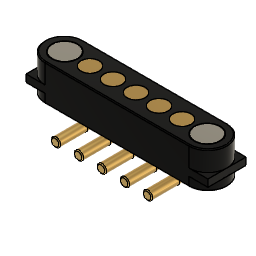
5359 Mag Connector (5-pin, Right Angle, Pads) (Autodesk Fusion 360 design; units mm, degrees)
Autodesk Fusion 360 part; units mm, degrees
sketch "Profile" plane through (0, 0, 0) normal (0, 0, 1) x (1, 0, 0)
  line L0 (-7.865, 0) -> (7.865, 0) construction
  line L1 (0, 2.1) -> (0, -2.1) construction
  circle A0 centre (-7.865, 0) radius 1.425
  line L2 (-10.04, 2.1) -> (10.04, 2.1)
  line L3 (10.04, 2.1) -> (10.04, -2.1)
  line L4 (10.04, -2.1) -> (-10.04, -2.1)
  line L5 (-10.04, -2.1) -> (-10.04, 2.1)
  circle A1 centre (-5.08, 0) radius 0.45
  circle A2 centre (-2.54, 0) radius 0.45
  circle A3 centre (0, 0) radius 0.45
  circle A4 centre (2.54, 0) radius 0.45
  circle A5 centre (5.08, 0) radius 0.45
  circle A6 centre (7.865, 0) radius 1.425
  arc A7 (-7.94, 2.1) -> (-7.94, -2.1) centre (-7.94, 0) ccw
  line L6 (-7.94, 2.1) -> (-7.94, -2.1) construction
  arc A8 (7.94, -2.1) -> (7.94, 2.1) centre (7.94, 0) ccw
  circle A9 centre (-5.08, 0) radius 0.5
  circle A10 centre (-5.08, 0) radius 1
  circle A11 centre (-2.54, 0) radius 0.5
  circle A12 centre (-2.54, 0) radius 1
  circle A13 centre (0, 0) radius 0.5
  circle A14 centre (0, 0) radius 1
  circle A15 centre (2.54, 0) radius 0.5
  circle A16 centre (2.54, 0) radius 1
  circle A17 centre (5.08, 0) radius 0.5
  circle A18 centre (5.08, 0) radius 1
  circle A19 centre (-5.08, 0) radius 0.575
  circle A20 centre (-2.54, 0) radius 0.575
  circle A21 centre (0, 0) radius 0.575
  circle A22 centre (2.54, 0) radius 0.575
  circle A23 centre (5.08, 0) radius 0.575
  dimension "d1" = 2.85
  dimension "d2" = 2.175
  dimension "d3" = 4.2
  dimension "d4" = 20.08
  dimension "d10" = 0.9
  dimension "d11" = 2.785
  dimension "d16" = 2.54
  dimension "d17" = 0
  dimension "d18" = 2.785
  dimension "d19" = 1
  dimension "d20" = 2
  dimension "d45" = 1.15
  constraint horizontal L0
  constraint coincident A3.centre L0
  constraint vertical L1
  constraint coincident L0 A0.centre
  constraint coincident L0.start A0.centre
  constraint horizontal L2
  constraint vertical L3
  constraint horizontal L4
  constraint vertical L5
  constraint symmetric L1 L3 L5
  constraint coincident L1.start L2
  constraint coincident L1.end L4
  constraint coincident L0 A1.centre
  constraint symmetric L1 A0 A6
  constraint coincident L2 A7.start
  constraint vertical L6
  constraint coincident L4 A7.end
  constraint coincident A7.centre L6
  constraint tangent L5 A7
  constraint symmetric L1 A7.start A8.end
  constraint symmetric L1 A7.end A8.start
  constraint symmetric L1 A7 A8
  constraint concentric A1 A9
  constraint concentric A1 A10
  constraint midpoint A3.centre L1
  constraint midpoint L0 A3.centre
  constraint concentric A10 A19
  measures "d1" diameter of A0
  measures "d2" distance of L0.start L5
  measures "d3" distance of L2.start L4.end
  measures "d4" distance of L2.start L2.end
  measures "d10" diameter of A1
  measures "d11" distance of L0.start A1.centre
  measures "d18" distance of A5.centre L0.end
  measures "d19" diameter of A9
  measures "d20" diameter of A10
  measures "d45" diameter of A19
extrude "Extrude - Housing" add sketch "Profile" along normal blind 4 contours L2 L4 A7 A8 makes body 1
extrude "Extrude - Housing Tabs" add sketch "Profile" along normal blind 0.8 from surface at 1 contours L2 L5 A7 | L4 L5 A7 | L2 L3 A8 | L3 L4 A8 bodies 1
fillet "Fillet - Housing Edges" radius 0.1 8 edges at (0, -2.1, 4) (10.04, 0, 4) (0, 2.1, 4) (-10.04, 0, 4) (0, -2.1, 0) (10.04, 0, 0) (0, 2.1, 0) (-10.04, 0, 0) on bodies 1
extrude "Extrude - Housing Pin Clearance" add sketch "Profile" along normal up to surface (3.8 mm away) from surface at 0.2 contours A10 | A12 | A14 | A16 | A18 bodies 1
copy_body "Body->Comp1" bodies 1 removing the originals makes body 2 in component "Housing"
extrude "Extrude - Magnets" add sketch "Profile" along normal blind 4 separate body contours A0 | A6 makes body 3 at (-6.4418, -0.071, 2.6667) makes body 4 at (9.2882, -0.071, 2.6667)
copy_body "Body->Comp2" bodies 3 removing the originals makes body 5 in component "Magnet"
fillet "Fillet - Magnets" radius 0.05 2 edges at (6.5364, -0.5153, 4) (6.5364, -0.5153, 0) on bodies 4
fillet "Fillet1" radius 0.05 2 edges at (-9.1936, -0.5153, 4) (-9.1936, -0.5153, 0) on bodies 5 in component "Magnet"
copy_body "CutPasteBodies1" bodies 4 removing the originals makes body 6 in component "Magnet"
extrude "Extrude - Pin Bottom" add sketch "Profile" against normal blind 0.1 separate body contours A1 | A9 makes body 7 in component "Pins"
extrude "Extrude - Pin Base" add sketch "Profile" along normal blind 0.2 contours A1 | A9 | A10 | A19 bodies 7 in component "Pins"
extrude "Extrude - Pin Body" add sketch "Profile" along normal blind 3.6 contours A9 | A19 bodies 7 in component "Pins"
ref_plane "WorkPlane1" through (-5.08, 0, 0) normal (1, 0, 0) x (0, 1, 0)
sketch "Pin Right Angle Profile" plane through (-5.08, 0, 0) normal (1, 0, 0) x (0, 1, 0)
  line L0 (-2, 4) -> (2, 4)
  line L1 (-2.1, 0.1) -> (-2.1, 1)
  line L2 (0, 0) -> (0, -0.65)
  line L3 (0, -0.65) -> (-0.75, -0.65) construction
  line L4 (-0.75, -0.65) -> (-0.75, -1.4) construction
  line L5 (-0.75, -1.4) -> (-3.85, -1.4)
  arc A0 (-0.75, -1.4) -> (0, -0.65) centre (-0.75, -0.65) ccw
  dimension "d92" = 5.4
  dimension "d93" = 1.75
  dimension "d94" = 0.75
  constraint vertical L2
  constraint perpendicular L2 L3
  constraint perpendicular L3 L4
  constraint perpendicular L4 L5
  constraint coincident L2.start origin
  constraint coincident L3.end L4.start
  constraint coincident L4.end L5.start
  measures "d92" distance of L0 L5
  measures "d93" distance of L1 L5.end
  measures "d94" distance of L2.end L3.end
sweep "Sweep - Pin Right Angle" add 1 faces at (-5.2393, 0.0491, -0.1) path "Pin Right Angle Profile" along L2 A0 L5 on bodies 7 bodies 7 in component "Pins"
fillet "Fillet - Pin" radius 0.1 1 edges at (-5.5462, -3.85, -1.5808) on bodies 7 in component "Pins"
extrude "Extrude - Pad Clearance" cut sketch "Profile" against normal up to surface (0.4 mm away) from surface at 4 contours A10 bodies 2 in component "Housing"
pattern_linear "R-Pattern - Pad Clearance" count 5 spacing 2.54 along (1, 0, 0) of "Extrude - Pad Clearance" in component "Housing"
extrude "Extrude - Pad" add sketch "Profile" along normal up to surface (0.4 mm away) from surface at 3.6 contours A1 | A9 | A10 | A19 bodies 7 in component "Pins"
pattern_linear "R-Pattern - Pads" count 5 spacing 2.54 along (1, 0, 0) of bodies 7 makes body 8 at (-1.9679, 0.0573, 1.3333) makes body 9 at (0.5721, 0.0573, 1.3333) makes body 10 at (3.1121, 0.0573, 1.3333) makes body 11 at (5.6521, 0.0573, 1.3333) in component "Pins"
component "Housing" placed x (1, 0, 0) y (0, 1, 0) z (0, 0, 1) at (0, 0, 0)
component "Magnet" placed x (1, 0, 0) y (0, 1, 0) z (0, 0, 1) at (0, 0, 0)
component "Pins" placed x (1, 0, 0) y (0, 1, 0) z (0, 0, 1) at (0, 0, 0)
equation "d89 = -( ( 2.54 * 2 ) * 1 mm )"
named bodies: "Housing", "Magnet", "Magnet (1)", "Magnet (2)", "Pin (1)", "Pin (2)", "Pin (3)", "Pin (4)", "Pin (5)"
